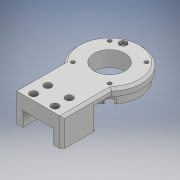
# Autodesk Inventor part: base_stepper
Saved by Autodesk Inventor 2017 (Build 210142000, 142)
## iProperties
Created: 2021-02-25
Part Number: base_stepper
Material: Generic
Document SubType Name: Modeling
Designer: paulg
Density: 1 g/cm^3
Appearance: Default
Author: paulg
Autodesk Inventor part; units mm, degrees
ref_plane "YZ Plane" through (0, 0, 0) normal (1, 0, 0) x (0, 1, 0)
ref_plane "XZ Plane" through (0, 0, 0) normal (0, 1, 0) x (-1, 0, 0)
ref_plane "XY Plane" through (0, 0, 0) normal (0, 0, 1) x (1, 0, 0)
sketch "Sketch1" plane through (0, 0, 0) normal (0, 0, 1) x (1, 0, 0)
  circle A0 centre (0, 0) radius 13
  circle A1 centre (0, 0) radius 25
  dimension "d0" = 50
  dimension "d1" = 26
  constraints: 2 centre point, 2 coincident
  measures "d0" diameter of A1
  measures "d1" diameter of A0
extrude "Extrusion1" add sketch "Sketch1" along normal blind 7
sketch "Sketch2" plane through (0, 0, 7) normal (0, 0, 1) x (1, 0, 0)
  circle A0 centre (0, 0) radius 13 projected
  circle A1 centre (0, 0) radius 25 projected
  circle A2 centre (0, 0) radius 27
  dimension "d4" = 2
  constraints: 1 centre point
  measures "d4" radial gap between concentric circles of A1 A2
extrude "Extrusion2" add sketch "Sketch2" along normal blind 1 contours A1 | A2
sketch "Sketch3" plane through (0, 0, 8) normal (0, 0, 1) x (1, 0, 0)
  circle A0 centre (0, 0) radius 13 projected
  circle A1 centre (0, 0) radius 27 projected
  line L0 (0, 0) -> (0, -39.0692) construction
  circle A2 centre (0, 0) radius 27 projected
  line L1 (20, -60) -> (-20, -60)
  line L2 (-20, -60) -> (-20, -18.1384)
  line L3 (-20, -18.1384) -> (20, -18.1384) construction
  line L4 (20, -18.1384) -> (20, -60)
  line L5 (20, -60) -> (-20, -18.1384) construction
  line L6 (-20, -60) -> (20, -18.1384) construction
  arc A3 (-20, -18.1384) -> (20, -18.1384) centre (0, 0) ccw
  dimension "d7" = 40
  dimension "d8" = 60
  constraints: 14 end point, 2 midpoint, 2 parallel, 2 point on circle, 1 centre point, 1 coincident, 1 horizontal, 1 perpendicular, 1 vertical, 4 other
  measures "d7" distance of L1.start L1.end
  measures "d8" distance from line of L1 point (0, 0)
extrude "Extrusion3" add sketch "Sketch3" along normal blind 5
sketch "Sketch4" plane through (0, 0, 0) normal (0, 0, -1) x (-1, 0, 0)
  circle A0 centre (0, 0) radius 13 projected
  circle A1 centre (0, 0) radius 25 projected
  line L0 (15.5, -15.5) -> (-15.5, -15.5) construction
  line L1 (-15.5, -15.5) -> (-15.5, 15.5) construction
  line L2 (-15.5, 15.5) -> (15.5, 15.5) construction
  line L3 (15.5, 15.5) -> (15.5, -15.5) construction
  line L4 (15.5, -15.5) -> (-15.5, 15.5) construction
  line L5 (-15.5, -15.5) -> (15.5, 15.5) construction
  dimension "d11" = 31
  constraints: 12 end point, 4 coincident, 2 midpoint, 2 parallel, 2 perpendicular, 1 horizontal
  measures "d11" distance of L2.end L0.start
hole "Hole1" at (15.5, 15.5, 0) at (-15.5, 15.5, 0) at (-15.5, -15.5, 0) at (15.5, -15.5, 0) direction (0, 0, 1) diameter 3.2 end through all counterbore diameter 6.2 counterbore depth 4
fillet "Fillet1" radius 1 8 edges at (17.4081, 17.9432, 2) (17.9432, 17.4081, 2) (-17.4081, 17.9432, 2) (-17.9432, 17.4081, 2) (-17.9432, -17.4081, 2) (-17.4081, -17.9432, 2) (17.9432, -17.4081, 2) (17.4081, -17.9432, 2)
sketch "Sketch5" plane through (0, 0, 0) normal (0, 0, -1) x (-1, 0, 0)
  arc A0 (-14.4888, -18.4304) -> (-14.7527, -20.1831) centre (-14.1626, -19.3758) ccw projected
  arc A1 (-14.7527, -20.1831) -> (14.7527, -20.1831) centre (0, 0) ccw projected
  arc A2 (14.7527, -20.1831) -> (14.4888, -18.4304) centre (14.1626, -19.3758) ccw projected
  arc A3 (18.4304, -14.4888) -> (14.4888, -18.4304) centre (15.5, -15.5) ccw projected
  arc A4 (18.4304, -14.4888) -> (20.1831, -14.7527) centre (19.3758, -14.1626) ccw projected
  arc A5 (20.1831, -14.7527) -> (20.1831, 14.7527) centre (0, 0) ccw projected
  arc A6 (20.1831, 14.7527) -> (18.4304, 14.4888) centre (19.3758, 14.1626) ccw projected
  arc A7 (14.4888, 18.4304) -> (18.4304, 14.4888) centre (15.5, 15.5) ccw projected
  arc A8 (14.4888, 18.4304) -> (14.7527, 20.1831) centre (14.1626, 19.3758) ccw projected
  arc A9 (14.7527, 20.1831) -> (-14.7527, 20.1831) centre (0, 0) ccw projected
  arc A10 (-14.7527, 20.1831) -> (-14.4888, 18.4304) centre (-14.1626, 19.3758) ccw projected
  arc A11 (-18.4304, 14.4888) -> (-14.4888, 18.4304) centre (-15.5, 15.5) ccw projected
  arc A12 (-18.4304, 14.4888) -> (-20.1831, 14.7527) centre (-19.3758, 14.1626) ccw projected
  arc A13 (-20.1831, 14.7527) -> (-20.1831, -14.7527) centre (0, 0) ccw projected
  arc A14 (-20.1831, -14.7527) -> (-18.4304, -14.4888) centre (-19.3758, -14.1626) ccw projected
  arc A15 (-14.4888, -18.4304) -> (-18.4304, -14.4888) centre (-15.5, -15.5) ccw projected
  circle A16 centre (0, 0) radius 13 projected
  line L0 (0, 0) -> (0, 21) construction
  circle A17 centre (0, 0) radius 21 construction
  line L1 (0, 0) -> (8.0364, 19.4015) construction
  point P0 (-8.0364, 19.4015)
  point P1 (-19.4015, 8.0364)
  point P2 (-19.4015, -8.0364)
  point P3 (-8.0364, -19.4015)
  point P4 (8.0364, -19.4015)
  point P5 (19.4015, -8.0364)
  point P6 (19.4015, 8.0364)
  dimension "d20" = 22.5
  dimension "d23" = 360
  dimension "d25" = 42
  constraints: 4 end point, 2 coincident, 2 point on circle, 1 centre point, 1 vertical, 9 other
  measures "d20" angle of L1 L0
  measures "d25" diameter of A17
hole "Hole2" at (-8.0364, 19.4015, 0) at (8.0364, 19.4015, 0) at (19.4015, 8.0364, 0) at (19.4015, -8.0364, 0) at (8.0364, -19.4015, 0) at (-8.0364, -19.4015, 0) at (-19.4015, -8.0364, 0) at (-19.4015, 8.0364, 0) direction (0, 0, 1) diameter 3.2 depth 6 tip angle 118
sketch "Sketch6" plane through (0, 0, 8) normal (0, 0, -1) x (-1, 0, 0)
  arc A0 (-20, -18.1384) -> (20, -18.1384) centre (0, 0) ccw projected
  line L0 (-20, -18.1384) -> (-20, -60) projected
  line L1 (-20, -60) -> (20, -60) projected
  line L2 (20, -60) -> (20, -18.1384) projected
  line L3 (-20, -18.1384) -> (-20, -60) projected
  arc A1 (-20, -29.9333) -> (20, -29.9333) centre (0, 0) ccw
  dimension "d33" = 36
  constraints: 2 point on circle, 2 point on line, 1 centre point, 1 coincident
  measures "d33" radius of A1
extrude "Extrusion4" add sketch "Sketch6" along normal blind 19 contours A1 L2 L1 L0
sketch "Sketch7" plane through (-20, -60, 13) normal (0, -1, 0) x (1, 0, 0)
  line L0 (40, -24) -> (40, 0) projected
  line L1 (0, 0) -> (40, 0) projected
  line L2 (0, 0) -> (0, -24) projected
  line L3 (40, -24) -> (0, -24) projected
  line L4 (40, -24) -> (0, -24) projected
  line L5 (20, -24) -> (20, -24.5)
  line L6 (32.8, -37.2) -> (7.2, -37.2)
  line L7 (7.2, -37.2) -> (7.2, -11.8)
  line L8 (7.2, -11.8) -> (32.8, -11.8)
  line L9 (32.8, -11.8) -> (32.8, -37.2)
  line L10 (32.8, -37.2) -> (7.2, -11.8) construction
  line L11 (7.2, -37.2) -> (32.8, -11.8) construction
  line L12 (7.2056, -12.5099) -> (7.9099, -11.8)
  line L13 (7.9099, -11.8) -> (7.1944, -11.0901)
  line L14 (7.1944, -11.0901) -> (6.4901, -11.8)
  line L15 (6.4901, -11.8) -> (7.2056, -12.5099)
  line L16 (7.2056, -12.5099) -> (7.1944, -11.0901) construction
  line L17 (7.9099, -11.8) -> (6.4901, -11.8) construction
  line L18 (32.8, -12.5071) -> (32.0929, -11.8)
  line L19 (32.0929, -11.8) -> (32.8, -11.0929)
  line L20 (32.8, -11.0929) -> (33.5071, -11.8)
  line L21 (33.5071, -11.8) -> (32.8, -12.5071)
  line L22 (32.8, -12.5071) -> (32.8, -11.0929) construction
  line L23 (32.0929, -11.8) -> (33.5071, -11.8) construction
  point P0 (20, -13)
  dimension "d36" = 25.6
  dimension "d37" = 25.4
  dimension "d38" = 0.5
  dimension "d39" = 1
  constraints: 38 end point, 7 midpoint, 6 parallel, 4 perpendicular, 3 horizontal, 2 equal length, 1 vertical
  measures "d36" distance of L7.end L8.end
  measures "d37" distance of L8.end L6.start
  measures "d38" distance of L5.start L5.end
  measures "d39" distance of L13.end L14.end
extrude "Extrusion5" cut sketch "Sketch7" against normal blind 22 contours L9 L6 L7 L3 | L3 L7 L15 L12 L8 L18 L9 | L18 L8 L9 | L9 L8 L19 L20 L21 | L15 L14 L13 L8 L7 | L7 L8 L12 L15
fillet "Fillet2" radius 2 2 edges at (-20, -29.9333, -1.5) (20, -29.9333, -1.5)
sketch "Sketch8" plane through (0, 0, 13) normal (0, 0, 1) x (1, 0, 0)
  circle A0 centre (-15.5, -15.5) radius 1.6 projected
  circle A1 centre (15.5, 15.5) radius 1.6 projected
  circle A2 centre (-15.5, 15.5) radius 1.6 projected
  circle A3 centre (15.5, -15.5) radius 1.6 projected
  circle A4 centre (0, 0) radius 13 projected
  line L0 (-20, -60) -> (20, -60) projected
  line L1 (20, -60) -> (20, -18.1384) projected
  arc A5 (20, -18.1384) -> (-20, -18.1384) centre (0, 0) ccw projected
  line L2 (-20, -18.1384) -> (-20, -60) projected
  line L3 (-12.0901, -38) -> (-12.0901, -60) projected
  line L4 (-12.0901, -38) -> (12.0929, -38) projected
  line L5 (12.0929, -60) -> (12.0929, -38) projected
  line L6 (-12.0901, -60) -> (12.0929, -60) projected
  line L7 (0, 0) -> (0.0014, -60)
  line L8 (-12.0901, -60) -> (12.0929, -60) projected
  line L9 (9.0011, -43) -> (-8.9989, -43) construction
  line L10 (-8.9989, -43) -> (-8.9989, -55) construction
  line L11 (-8.9989, -55) -> (9.0011, -55) construction
  line L12 (9.0011, -55) -> (9.0011, -43) construction
  line L13 (9.0011, -43) -> (-8.9989, -55) construction
  line L14 (-8.9989, -43) -> (9.0011, -55) construction
  point P0 (0.0011, -49)
  dimension "d43" = 18
  dimension "d44" = 5
  dimension "d45" = 5
  constraints: 14 end point, 3 coincident, 3 midpoint, 2 parallel, 1 horizontal, 1 perpendicular, 1 point on line
  measures "d43" distance of L10.end L11.end
  measures "d44" distance between parallel lines of L11 L0
  measures "d45" distance between parallel lines of L4 L9
hole "Hole3" at (-8.9989, -43, 13) at (-8.9989, -55, 13) at (9.0011, -43, 13) at (9.0011, -55, 13) direction (0, 0, -1) diameter 3.2 end through all counterbore diameter 6.2 counterbore depth 7
chamfer "Chamfer1" distance 1.5 angle 45 4 edges at (-8.9989, -39.9, 6) (-8.9989, -51.9, 6) (9.0011, -51.9, 6) (9.0011, -39.9, 6)
chamfer "Chamfer2" distance 2 angle 45 2 edges at (20, -39.0692, 13) (-20, -39.0692, 13)
chamfer "Chamfer3" distance 2 angle 45 3 edges at (19.0259, -19.1576, 13) (-19.0259, -19.1576, 13) (0, 27, 13)
chamfer "Chamfer4" distance 2 angle 45 2 edges at (20, -60, 0) (-20, -60, 0)
sketch "Sketch9" plane through (0, 0, 13) normal (0, 0, 1) x (1, 0, 0)
  circle A0 centre (-19.4015, -8.0364) radius 1.6 projected
  circle A1 centre (8.0364, -19.4015) radius 1.6 projected
  circle A2 centre (19.4015, 8.0364) radius 1.6 projected
  circle A3 centre (-8.0364, 19.4015) radius 1.6 projected
  circle A4 centre (8.0364, 19.4015) radius 1.6 projected
  circle A5 centre (19.4015, -8.0364) radius 1.6 projected
  circle A6 centre (-8.0364, -19.4015) radius 1.6 projected
  circle A7 centre (-19.4015, 8.0364) radius 1.6 projected
  arc A8 (14.7527, -20.1831) -> (14.4888, -18.4304) centre (14.1626, -19.3758) ccw projected
  arc A9 (-14.7527, -20.1831) -> (14.7527, -20.1831) centre (0, 0) ccw projected
  arc A10 (-14.4888, -18.4304) -> (-14.7527, -20.1831) centre (-14.1626, -19.3758) ccw projected
  arc A11 (-14.4888, -18.4304) -> (-18.4304, -14.4888) centre (-15.5, -15.5) ccw projected
  arc A12 (-20.1831, -14.7527) -> (-18.4304, -14.4888) centre (-19.3758, -14.1626) ccw projected
  arc A13 (-20.1831, 14.7527) -> (-20.1831, -14.7527) centre (0, 0) ccw projected
  arc A14 (-18.4304, 14.4888) -> (-20.1831, 14.7527) centre (-19.3758, 14.1626) ccw projected
  arc A15 (-18.4304, 14.4888) -> (-14.4888, 18.4304) centre (-15.5, 15.5) ccw projected
  arc A16 (-14.7527, 20.1831) -> (-14.4888, 18.4304) centre (-14.1626, 19.3758) ccw projected
  arc A17 (14.7527, 20.1831) -> (-14.7527, 20.1831) centre (0, 0) ccw projected
  arc A18 (14.4888, 18.4304) -> (14.7527, 20.1831) centre (14.1626, 19.3758) ccw projected
  arc A19 (14.4888, 18.4304) -> (18.4304, 14.4888) centre (15.5, 15.5) ccw projected
  arc A20 (20.1831, 14.7527) -> (18.4304, 14.4888) centre (19.3758, 14.1626) ccw projected
  arc A21 (20.1831, -14.7527) -> (20.1831, 14.7527) centre (0, 0) ccw projected
  arc A22 (18.4304, -14.4888) -> (20.1831, -14.7527) centre (19.3758, -14.1626) ccw projected
  arc A23 (18.4304, -14.4888) -> (14.4888, -18.4304) centre (15.5, -15.5) ccw projected
  circle A24 centre (0, 0) radius 13 projected
  circle A25 centre (-8.0364, 19.4015) radius 1.6 projected
  line L0 (-11.0234, 18.1642) -> (-10.6014, 21.3697)
  line L1 (-10.6014, 21.3697) -> (-7.6143, 22.607)
  line L2 (-7.6143, 22.607) -> (-5.0493, 20.6387)
  line L3 (-5.0493, 20.6387) -> (-5.4713, 17.4332)
  line L4 (-5.4713, 17.4332) -> (-8.4584, 16.196)
  line L5 (-8.4584, 16.196) -> (-11.0234, 18.1642)
  line L6 (0, 0) -> (-8.0364, 19.4015)
  dimension "d65" = 5.6
  constraints: 14 end point, 1 coincident, 1 perpendicular, 13 other
  measures "d65" distance between parallel lines of L4 L1
extrude "Extrusion6" cut sketch "Sketch9" against normal blind 3 contours A3 | L0 L1 L2 L3 L4 L5
body "Solid1"
